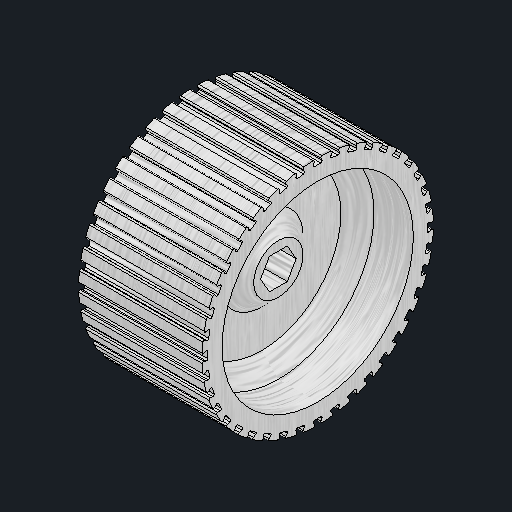
# Autodesk Inventor part: PLATE,FLYWHEEL,HUB
Saved by Autodesk Inventor 2026.1 (Build 301233020, 233B)
## iProperties
Created: 2026-02-01
Part Number: PLATE,FLYWHEEL,HUB
Material: Aluminum 7075
Document SubType Name: Modeling
Designer: Owen L
Mass: 390.303 g
Surface Area: 495.556 cm^2
Volume: 138.898 cm^3
Density: 2.81 g/cm^3
Appearance: Satin - Brushed Heavy
Author: Owen L
Autodesk Inventor part; units mm, degrees
ref_plane "YZ Plane" through (0, 0, 0) normal (1, 0, 0) x (0, 1, 0)
ref_plane "XZ Plane" through (0, 0, 0) normal (0, 1, 0) x (-1, 0, 0)
ref_plane "XY Plane" through (0, 0, 0) normal (0, 0, 1) x (1, 0, 0)
sketch "Sketch1" plane through (0, 0, 0) normal (0, 0, 1) x (1, 0, 0)
  line L0 (0, -9.525) -> (0, 57.15) projected
  line L1 (-35.56, 0) -> (35.56, 0) projected
  line L2 (-9.2075, 0) -> (-9.2075, 10.16)
  line L3 (-9.2075, 10.16) -> (-2.3812, 16.9863)
  line L4 (-2.3812, 16.9863) -> (-2.3813, 32.5438)
  line L5 (-2.3813, 32.5438) -> (-9.2075, 39.37)
  line L6 (-9.2075, 39.37) -> (-25.4, 39.37)
  line L7 (-25.4, 39.37) -> (-25.4, 47.625)
  line L8 (-25.4, 47.625) -> (0, 47.625)
  line L9 (9.2075, 0) -> (9.2075, 10.16)
  line L10 (9.2075, 10.16) -> (2.3812, 16.9863)
  line L11 (2.3812, 16.9863) -> (2.3813, 32.5438)
  line L12 (2.3813, 32.5438) -> (9.2075, 39.37)
  line L13 (9.2075, 39.37) -> (25.4, 39.37)
  line L14 (25.4, 39.37) -> (25.4, 47.625)
  line L15 (25.4, 47.625) -> (0, 47.625)
  point P0 (0, 0)
  dimension "d0" = 10.16
  dimension "d1" = 18.415
  dimension "d3" = 4.7625
  dimension "d4" = 45
  dimension "d5" = 45
  dimension "d6" = 50.8
  dimension "d7" = 8.255
  dimension "d8" = 95.25
  constraints: 28 end point, 7 symmetric about line, 4 perpendicular, 2 point on line, 2 vertical
  measures "d0" distance of L2.start L2.end
  measures "d1" diameter of L2 L0
  measures "d3" diameter of L4 L0
  measures "d4" angle of L1 L3
  measures "d5" angle of L5 L1
  measures "d6" diameter of L7 L0
  measures "d7" distance of L6.end L7.end
  measures "d8" diameter of L8 L1
revolve "Revolution1" add sketch "Sketch1" angle 360 about axis through (-10, 0, 0) along (1, 0, 0)
sketch "Sketch2" plane through (-9.2075, 0, 0) normal (-1, 0, 0) x (0, 0, 1)
  circle A0 centre (0, 0) radius 16.9863 projected
  line L0 (7.3323, 0) -> (3.6662, -6.35)
  line L1 (3.6662, -6.35) -> (-3.6662, -6.35)
  line L2 (-3.6662, -6.35) -> (-7.3323, 0)
  line L3 (-7.3323, 0) -> (-3.6662, 6.35)
  line L4 (-3.6662, 6.35) -> (3.6662, 6.35)
  line L5 (3.6662, 6.35) -> (7.3323, 0)
  dimension "d10" = 12.7
  constraints: 12 end point, 1 coincident, 1 horizontal, 13 other
  measures "d10" distance between parallel lines of L4 L1
extrude "Extrusion1" cut sketch "Sketch2" against normal through all contours L0 L1 L2 L3 L4 L5
sketch "Sketch3" plane through (-25.4, 0, 0) normal (-1, 0, 0) x (0, 0, 1)
  circle A0 centre (0, 0) radius 47.625 projected
  line L0 (-1.016, 47.6142) -> (-2.0955, 45.212)
  line L1 (1.016, 47.6142) -> (2.0955, 45.212)
  line L2 (2.0955, 45.212) -> (-2.0955, 45.212)
  point P0 (0, 45.212)
  dimension "d13" = 4.191
  dimension "d14" = 2.413
  dimension "d15" = 2.032
  constraints: 6 end point, 2 point on circle, 1 equal length, 1 horizontal, 1 midpoint, 1 vertical alignment
  measures "d13" distance of L1.end L0.end
  measures "d14" distance edge to line of A0 L2
  measures "d15" distance of L1.start L0.start
extrude "Extrusion2" cut sketch "Sketch3" against normal through all contours L1 L2 L0 A0 picked at (0.1129, 46.0159)
fillet "Fillet1" radius 0.508 4 edges at (0, 45.212, 2.0955) (0, 45.212, -2.0955) (0, 47.6142, 1.016) (0, 47.6142, -1.016)
pattern_circular "Circular Pattern1" count 40 over 360 about axis through (0, 0, 0) along (1, 0, 0) of "Extrusion2", "Fillet1"
sketch "WaterJet Profile" plane through (0, 0, 0) normal (1, 0, 0) x (0, 1, 0)
  line L0 (55, 55) -> (-55, 55)
  line L1 (-55, 55) -> (-55, -55)
  line L2 (-55, -55) -> (55, -55)
  line L3 (55, -55) -> (55, 55)
  line L4 (55, 55) -> (-55, -55) construction
  line L5 (-55, 55) -> (55, -55) construction
  point P0 (0, 0)
  dimension "d28" = 110
  dimension "d29" = 110
  constraints: 12 end point, 2 midpoint, 2 parallel, 1 horizontal, 1 perpendicular
  measures "d28" distance of L2.end L1.end
  measures "d29" distance of L1.end L0.end
sketch "EDM Profile" plane through (0, 0, 0) normal (1, 0, 0) x (0, 1, 0)
  arc A0 (45.212, -1.3103) -> (45.9282, -1.7736) centre (45.72, -1.3103) ccw projected
  line L0 (45.9282, -1.7736) -> (46.8739, -1.3487) projected
  arc A1 (47.5898, -1.8316) -> (46.8739, -1.3487) centre (47.0821, -1.812) ccw projected
  arc A2 (47.2904, -5.6357) -> (47.5898, -1.8316) centre (0, 0) ccw projected
  arc A3 (46.5078, -6.0006) -> (47.2904, -5.6357) centre (46.7859, -5.5756) ccw projected
  line L1 (46.5078, -6.0006) -> (45.6402, -5.433) projected
  arc A4 (45.6402, -5.433) -> (44.8603, -5.7786) centre (45.3621, -5.858) ccw projected
  line L2 (44.8603, -5.7786) -> (44.4504, -8.3669) projected
  arc A5 (44.4504, -8.3669) -> (45.0853, -8.9366) centre (44.9521, -8.4463) ccw projected
  line L3 (45.0853, -8.9366) -> (46.0858, -8.6647) projected
  arc A6 (46.7173, -9.2537) -> (46.0858, -8.6647) centre (46.219, -9.155) ccw projected
  arc A7 (45.8265, -12.9641) -> (46.7173, -9.2537) centre (0, 0) ccw projected
  arc A8 (44.9965, -13.2022) -> (45.8265, -12.9641) centre (45.3377, -12.8258) ccw projected
  line L4 (44.9965, -13.2022) -> (44.2284, -12.5058) projected
  arc A9 (44.2284, -12.5058) -> (43.4041, -12.7251) centre (43.8872, -12.8821) ccw projected
  line L5 (43.4041, -12.7251) -> (42.5943, -15.2174) projected
  arc A10 (42.5943, -15.2174) -> (43.1323, -15.8794) centre (43.0774, -15.3744) ccw projected
  line L6 (43.1323, -15.8794) -> (44.163, -15.7675) projected
  arc A11 (44.6946, -16.448) -> (44.163, -15.7675) centre (44.2178, -16.2725) ccw projected
  arc A12 (43.2343, -19.9734) -> (44.6946, -16.448) centre (0, 0) ccw projected
  arc A13 (42.3772, -20.0786) -> (43.2343, -19.9734) centre (42.7731, -19.7603) ccw projected
  line L7 (42.3772, -20.0786) -> (41.7276, -19.2707) projected
  arc A14 (41.7276, -19.2707) -> (40.879, -19.3584) centre (41.3317, -19.589) ccw projected
  line L8 (40.879, -19.3584) -> (39.6893, -21.6933) projected
  arc A15 (39.6893, -21.6933) -> (40.1171, -22.4313) centre (40.142, -21.9239) ccw projected
  line L9 (40.1171, -22.4313) -> (41.1527, -22.482) projected
  arc A16 (41.5713, -23.2372) -> (41.1527, -22.482) centre (41.1279, -22.9894) ccw projected
  arc A17 (39.5775, -26.4908) -> (41.5713, -23.2372) centre (0, 0) ccw projected
  arc A18 (38.7145, -26.4607) -> (39.5775, -26.4908) centre (39.1553, -26.2082) ccw projected
  line L10 (38.7145, -26.4607) -> (38.1992, -25.561) projected
  arc A19 (38.1992, -25.561) -> (37.3474, -25.5149) centre (37.7584, -25.8135) ccw projected
  line L11 (37.3474, -25.5149) -> (35.8071, -27.635) projected
  arc A20 (35.8071, -27.635) -> (36.1142, -28.4308) centre (36.2181, -27.9336) ccw projected
  line L12 (36.1142, -28.4308) -> (37.1291, -28.6429) projected
  arc A21 (37.4244, -29.4543) -> (37.1291, -28.6429) centre (37.0252, -29.1401) ccw projected
  arc A22 (34.9462, -32.3559) -> (37.4244, -29.4543) centre (0, 0) ccw projected
  arc A23 (34.0985, -32.1912) -> (34.9462, -32.3559) centre (34.5734, -32.0108) ccw projected
  line L13 (34.0985, -32.1912) -> (33.7303, -31.222) projected
  arc A24 (33.7303, -31.222) -> (32.8962, -31.0432) centre (33.2554, -31.4024) ccw projected
  line L14 (32.8962, -31.0432) -> (31.0432, -32.8962) projected
  arc A25 (31.0432, -32.8962) -> (31.222, -33.7303) centre (31.4024, -33.2554) ccw projected
  line L15 (31.222, -33.7303) -> (32.1912, -34.0985) projected
  arc A26 (32.3559, -34.9462) -> (32.1912, -34.0985) centre (32.0108, -34.5734) ccw projected
  arc A27 (29.4543, -37.4244) -> (32.3559, -34.9462) centre (0, 0) ccw projected
  arc A28 (28.6429, -37.1291) -> (29.4543, -37.4244) centre (29.1401, -37.0252) ccw projected
  line L16 (28.6429, -37.1291) -> (28.4308, -36.1142) projected
  arc A29 (28.4308, -36.1142) -> (27.635, -35.8071) centre (27.9336, -36.2181) ccw projected
  line L17 (27.635, -35.8071) -> (25.5149, -37.3474) projected
  arc A30 (25.5149, -37.3474) -> (25.561, -38.1992) centre (25.8135, -37.7584) ccw projected
  line L18 (25.561, -38.1992) -> (26.4607, -38.7145) projected
  arc A31 (26.4908, -39.5775) -> (26.4607, -38.7145) centre (26.2082, -39.1553) ccw projected
  arc A32 (23.2372, -41.5713) -> (26.4908, -39.5775) centre (0, 0) ccw projected
  arc A33 (22.482, -41.1527) -> (23.2372, -41.5713) centre (22.9894, -41.1279) ccw projected
  line L19 (22.482, -41.1527) -> (22.4313, -40.1171) projected
  arc A34 (22.4313, -40.1171) -> (21.6933, -39.6893) centre (21.9239, -40.142) ccw projected
  line L20 (21.6933, -39.6893) -> (19.3584, -40.879) projected
  arc A35 (19.3584, -40.879) -> (19.2707, -41.7276) centre (19.589, -41.3317) ccw projected
  line L21 (19.2707, -41.7276) -> (20.0786, -42.3772) projected
  arc A36 (19.9734, -43.2343) -> (20.0786, -42.3772) centre (19.7603, -42.7731) ccw projected
  arc A37 (16.448, -44.6946) -> (19.9734, -43.2343) centre (0, 0) ccw projected
  arc A38 (15.7675, -44.163) -> (16.448, -44.6946) centre (16.2725, -44.2178) ccw projected
  line L22 (15.7675, -44.163) -> (15.8794, -43.1323) projected
  arc A39 (15.8794, -43.1323) -> (15.2174, -42.5943) centre (15.3744, -43.0774) ccw projected
  line L23 (15.2174, -42.5943) -> (12.7251, -43.4041) projected
  arc A40 (12.7251, -43.4041) -> (12.5058, -44.2284) centre (12.8821, -43.8872) ccw projected
  line L24 (12.5058, -44.2284) -> (13.2022, -44.9965) projected
  arc A41 (12.9641, -45.8265) -> (13.2022, -44.9965) centre (12.8258, -45.3377) ccw projected
  arc A42 (9.2537, -46.7173) -> (12.9641, -45.8265) centre (0, 0) ccw projected
  arc A43 (8.6647, -46.0858) -> (9.2537, -46.7173) centre (9.155, -46.219) ccw projected
  line L25 (8.6647, -46.0858) -> (8.9366, -45.0853) projected
  arc A44 (8.9366, -45.0853) -> (8.3669, -44.4504) centre (8.4463, -44.9521) ccw projected
  line L26 (8.3669, -44.4504) -> (5.7786, -44.8603) projected
  arc A45 (5.7786, -44.8603) -> (5.433, -45.6402) centre (5.858, -45.3621) ccw projected
  line L27 (5.433, -45.6402) -> (6.0006, -46.5078) projected
  arc A46 (5.6357, -47.2904) -> (6.0006, -46.5078) centre (5.5756, -46.7859) ccw projected
  arc A47 (1.8316, -47.5898) -> (5.6357, -47.2904) centre (0, 0) ccw projected
  arc A48 (1.3487, -46.8739) -> (1.8316, -47.5898) centre (1.812, -47.0821) ccw projected
  line L28 (1.3487, -46.8739) -> (1.7736, -45.9282) projected
  arc A49 (1.7736, -45.9282) -> (1.3103, -45.212) centre (1.3103, -45.72) ccw projected
  line L29 (1.3103, -45.212) -> (-1.3103, -45.212) projected
  arc A50 (-1.3103, -45.212) -> (-1.7736, -45.9282) centre (-1.3103, -45.72) ccw projected
  line L30 (-1.7736, -45.9282) -> (-1.3487, -46.8739) projected
  arc A51 (-1.8316, -47.5898) -> (-1.3487, -46.8739) centre (-1.812, -47.0821) ccw projected
  arc A52 (-5.6357, -47.2904) -> (-1.8316, -47.5898) centre (0, 0) ccw projected
  arc A53 (-6.0006, -46.5078) -> (-5.6357, -47.2904) centre (-5.5756, -46.7859) ccw projected
  line L31 (-6.0006, -46.5078) -> (-5.433, -45.6402) projected
  arc A54 (-5.433, -45.6402) -> (-5.7786, -44.8603) centre (-5.858, -45.3621) ccw projected
  line L32 (-5.7786, -44.8603) -> (-8.3669, -44.4504) projected
  arc A55 (-8.3669, -44.4504) -> (-8.9366, -45.0853) centre (-8.4463, -44.9521) ccw projected
  line L33 (-8.9366, -45.0853) -> (-8.6647, -46.0858) projected
  arc A56 (-9.2537, -46.7173) -> (-8.6647, -46.0858) centre (-9.155, -46.219) ccw projected
  arc A57 (-12.9641, -45.8265) -> (-9.2537, -46.7173) centre (0, 0) ccw projected
  arc A58 (-13.2022, -44.9965) -> (-12.9641, -45.8265) centre (-12.8258, -45.3377) ccw projected
  line L34 (-13.2022, -44.9965) -> (-12.5058, -44.2284) projected
  arc A59 (-12.5058, -44.2284) -> (-12.7251, -43.4041) centre (-12.8821, -43.8872) ccw projected
  line L35 (-12.7251, -43.4041) -> (-15.2174, -42.5943) projected
  arc A60 (-15.2174, -42.5943) -> (-15.8794, -43.1323) centre (-15.3744, -43.0774) ccw projected
  line L36 (-15.8794, -43.1323) -> (-15.7675, -44.163) projected
  arc A61 (-16.448, -44.6946) -> (-15.7675, -44.163) centre (-16.2725, -44.2178) ccw projected
  arc A62 (-19.9734, -43.2343) -> (-16.448, -44.6946) centre (0, 0) ccw projected
  arc A63 (-20.0786, -42.3772) -> (-19.9734, -43.2343) centre (-19.7603, -42.7731) ccw projected
  line L37 (-20.0786, -42.3772) -> (-19.2707, -41.7276) projected
  arc A64 (-19.2707, -41.7276) -> (-19.3584, -40.879) centre (-19.589, -41.3317) ccw projected
  line L38 (-19.3584, -40.879) -> (-21.6933, -39.6893) projected
  arc A65 (-21.6933, -39.6893) -> (-22.4313, -40.1171) centre (-21.9239, -40.142) ccw projected
  line L39 (-22.4313, -40.1171) -> (-22.482, -41.1527) projected
  arc A66 (-23.2372, -41.5713) -> (-22.482, -41.1527) centre (-22.9894, -41.1279) ccw projected
  arc A67 (-26.4908, -39.5775) -> (-23.2372, -41.5713) centre (0, 0) ccw projected
  arc A68 (-26.4607, -38.7145) -> (-26.4908, -39.5775) centre (-26.2082, -39.1553) ccw projected
  line L40 (-26.4607, -38.7145) -> (-25.561, -38.1992) projected
  arc A69 (-25.561, -38.1992) -> (-25.5149, -37.3474) centre (-25.8135, -37.7584) ccw projected
  line L41 (-25.5149, -37.3474) -> (-27.635, -35.8071) projected
  arc A70 (-27.635, -35.8071) -> (-28.4308, -36.1142) centre (-27.9336, -36.2181) ccw projected
  line L42 (-28.4308, -36.1142) -> (-28.6429, -37.1291) projected
  arc A71 (-29.4543, -37.4244) -> (-28.6429, -37.1291) centre (-29.1401, -37.0252) ccw projected
  arc A72 (-32.3559, -34.9462) -> (-29.4543, -37.4244) centre (0, 0) ccw projected
  arc A73 (-32.1912, -34.0985) -> (-32.3559, -34.9462) centre (-32.0108, -34.5734) ccw projected
  line L43 (-32.1912, -34.0985) -> (-31.222, -33.7303) projected
  arc A74 (-31.222, -33.7303) -> (-31.0432, -32.8962) centre (-31.4024, -33.2554) ccw projected
  line L44 (-31.0432, -32.8962) -> (-32.8962, -31.0432) projected
  arc A75 (-32.8962, -31.0432) -> (-33.7303, -31.222) centre (-33.2554, -31.4024) ccw projected
  line L45 (-33.7303, -31.222) -> (-34.0985, -32.1912) projected
  arc A76 (-34.9462, -32.3559) -> (-34.0985, -32.1912) centre (-34.5734, -32.0108) ccw projected
  arc A77 (-37.4244, -29.4543) -> (-34.9462, -32.3559) centre (0, 0) ccw projected
  arc A78 (-37.1291, -28.6429) -> (-37.4244, -29.4543) centre (-37.0252, -29.1401) ccw projected
  line L46 (-37.1291, -28.6429) -> (-36.1142, -28.4308) projected
  arc A79 (-36.1142, -28.4308) -> (-35.8071, -27.635) centre (-36.2181, -27.9336) ccw projected
  line L47 (-35.8071, -27.635) -> (-37.3474, -25.5149) projected
  arc A80 (-37.3474, -25.5149) -> (-38.1992, -25.561) centre (-37.7584, -25.8135) ccw projected
  line L48 (-38.1992, -25.561) -> (-38.7145, -26.4607) projected
  arc A81 (-39.5775, -26.4908) -> (-38.7145, -26.4607) centre (-39.1553, -26.2082) ccw projected
  arc A82 (-41.5713, -23.2372) -> (-39.5775, -26.4908) centre (0, 0) ccw projected
  arc A83 (-41.1527, -22.482) -> (-41.5713, -23.2372) centre (-41.1279, -22.9894) ccw projected
  line L49 (-41.1527, -22.482) -> (-40.1171, -22.4313) projected
  arc A84 (-40.1171, -22.4313) -> (-39.6893, -21.6933) centre (-40.142, -21.9239) ccw projected
  line L50 (-39.6893, -21.6933) -> (-40.879, -19.3584) projected
  arc A85 (-40.879, -19.3584) -> (-41.7276, -19.2707) centre (-41.3317, -19.589) ccw projected
  line L51 (-41.7276, -19.2707) -> (-42.3772, -20.0786) projected
  arc A86 (-43.2343, -19.9734) -> (-42.3772, -20.0786) centre (-42.7731, -19.7603) ccw projected
  arc A87 (-44.6946, -16.448) -> (-43.2343, -19.9734) centre (0, 0) ccw projected
  arc A88 (-44.163, -15.7675) -> (-44.6946, -16.448) centre (-44.2178, -16.2725) ccw projected
  line L52 (-44.163, -15.7675) -> (-43.1323, -15.8794) projected
  arc A89 (-43.1323, -15.8794) -> (-42.5943, -15.2174) centre (-43.0774, -15.3744) ccw projected
  line L53 (-42.5943, -15.2174) -> (-43.4041, -12.7251) projected
  arc A90 (-43.4041, -12.7251) -> (-44.2284, -12.5058) centre (-43.8872, -12.8821) ccw projected
  line L54 (-44.2284, -12.5058) -> (-44.9965, -13.2022) projected
  arc A91 (-45.8265, -12.9641) -> (-44.9965, -13.2022) centre (-45.3377, -12.8258) ccw projected
  arc A92 (-46.7173, -9.2537) -> (-45.8265, -12.9641) centre (0, 0) ccw projected
  arc A93 (-46.0858, -8.6647) -> (-46.7173, -9.2537) centre (-46.219, -9.155) ccw projected
  line L55 (-46.0858, -8.6647) -> (-45.0853, -8.9366) projected
  arc A94 (-45.0853, -8.9366) -> (-44.4504, -8.3669) centre (-44.9521, -8.4463) ccw projected
  line L56 (-44.4504, -8.3669) -> (-44.8603, -5.7786) projected
  arc A95 (-44.8603, -5.7786) -> (-45.6402, -5.433) centre (-45.3621, -5.858) ccw projected
  line L57 (-45.6402, -5.433) -> (-46.5078, -6.0006) projected
  arc A96 (-47.2904, -5.6357) -> (-46.5078, -6.0006) centre (-46.7859, -5.5756) ccw projected
  arc A97 (-47.5898, -1.8316) -> (-47.2904, -5.6357) centre (0, 0) ccw projected
  arc A98 (-46.8739, -1.3487) -> (-47.5898, -1.8316) centre (-47.0821, -1.812) ccw projected
  line L58 (-46.8739, -1.3487) -> (-45.9282, -1.7736) projected
  arc A99 (-45.9282, -1.7736) -> (-45.212, -1.3103) centre (-45.72, -1.3103) ccw projected
  line L59 (-45.212, -1.3103) -> (-45.212, 1.3103) projected
  arc A100 (-45.212, 1.3103) -> (-45.9282, 1.7736) centre (-45.72, 1.3103) ccw projected
  line L60 (-45.9282, 1.7736) -> (-46.8739, 1.3487) projected
  arc A101 (-47.5898, 1.8316) -> (-46.8739, 1.3487) centre (-47.0821, 1.812) ccw projected
  arc A102 (-47.2904, 5.6357) -> (-47.5898, 1.8316) centre (0, 0) ccw projected
  arc A103 (-46.5078, 6.0006) -> (-47.2904, 5.6357) centre (-46.7859, 5.5756) ccw projected
  line L61 (-46.5078, 6.0006) -> (-45.6402, 5.433) projected
  arc A104 (-45.6402, 5.433) -> (-44.8603, 5.7786) centre (-45.3621, 5.858) ccw projected
  line L62 (-44.8603, 5.7786) -> (-44.4504, 8.3669) projected
  arc A105 (-44.4504, 8.3669) -> (-45.0853, 8.9366) centre (-44.9521, 8.4463) ccw projected
  line L63 (-45.0853, 8.9366) -> (-46.0858, 8.6647) projected
  arc A106 (-46.7173, 9.2537) -> (-46.0858, 8.6647) centre (-46.219, 9.155) ccw projected
  arc A107 (-45.8265, 12.9641) -> (-46.7173, 9.2537) centre (0, 0) ccw projected
  arc A108 (-44.9965, 13.2022) -> (-45.8265, 12.9641) centre (-45.3377, 12.8258) ccw projected
  line L64 (-44.9965, 13.2022) -> (-44.2284, 12.5058) projected
  arc A109 (-44.2284, 12.5058) -> (-43.4041, 12.7251) centre (-43.8872, 12.8821) ccw projected
  line L65 (-43.4041, 12.7251) -> (-42.5943, 15.2174) projected
  arc A110 (-42.5943, 15.2174) -> (-43.1323, 15.8794) centre (-43.0774, 15.3744) ccw projected
  line L66 (-43.1323, 15.8794) -> (-44.163, 15.7675) projected
  arc A111 (-44.6946, 16.448) -> (-44.163, 15.7675) centre (-44.2178, 16.2725) ccw projected
  arc A112 (-43.2343, 19.9734) -> (-44.6946, 16.448) centre (0, 0) ccw projected
  arc A113 (-42.3772, 20.0786) -> (-43.2343, 19.9734) centre (-42.7731, 19.7603) ccw projected
  line L67 (-42.3772, 20.0786) -> (-41.7276, 19.2707) projected
  arc A114 (-41.7276, 19.2707) -> (-40.879, 19.3584) centre (-41.3317, 19.589) ccw projected
  line L68 (-40.879, 19.3584) -> (-39.6893, 21.6933) projected
  arc A115 (-39.6893, 21.6933) -> (-40.1171, 22.4313) centre (-40.142, 21.9239) ccw projected
  line L69 (-40.1171, 22.4313) -> (-41.1527, 22.482) projected
  arc A116 (-41.5713, 23.2372) -> (-41.1527, 22.482) centre (-41.1279, 22.9894) ccw projected
  arc A117 (-39.5775, 26.4908) -> (-41.5713, 23.2372) centre (0, 0) ccw projected
  arc A118 (-38.7145, 26.4607) -> (-39.5775, 26.4908) centre (-39.1553, 26.2082) ccw projected
  line L70 (-38.7145, 26.4607) -> (-38.1992, 25.561) projected
  arc A119 (-38.1992, 25.561) -> (-37.3474, 25.5149) centre (-37.7584, 25.8135) ccw projected
  line L71 (-37.3474, 25.5149) -> (-35.8071, 27.635) projected
  arc A120 (-35.8071, 27.635) -> (-36.1142, 28.4308) centre (-36.2181, 27.9336) ccw projected
  line L72 (-36.1142, 28.4308) -> (-37.1291, 28.6429) projected
  arc A121 (-37.4244, 29.4543) -> (-37.1291, 28.6429) centre (-37.0252, 29.1401) ccw projected
  arc A122 (-34.9462, 32.3559) -> (-37.4244, 29.4543) centre (0, 0) ccw projected
  arc A123 (-34.0985, 32.1912) -> (-34.9462, 32.3559) centre (-34.5734, 32.0108) ccw projected
  line L73 (-34.0985, 32.1912) -> (-33.7303, 31.222) projected
  arc A124 (-33.7303, 31.222) -> (-32.8962, 31.0432) centre (-33.2554, 31.4024) ccw projected
  line L74 (-32.8962, 31.0432) -> (-31.0432, 32.8962) projected
  arc A125 (-31.0432, 32.8962) -> (-31.222, 33.7303) centre (-31.4024, 33.2554) ccw projected
  line L75 (-31.222, 33.7303) -> (-32.1912, 34.0985) projected
  arc A126 (-32.3559, 34.9462) -> (-32.1912, 34.0985) centre (-32.0108, 34.5734) ccw projected
  arc A127 (-29.4543, 37.4244) -> (-32.3559, 34.9462) centre (0, 0) ccw projected
  arc A128 (-28.6429, 37.1291) -> (-29.4543, 37.4244) centre (-29.1401, 37.0252) ccw projected
  line L76 (-28.6429, 37.1291) -> (-28.4308, 36.1142) projected
  arc A129 (-28.4308, 36.1142) -> (-27.635, 35.8071) centre (-27.9336, 36.2181) ccw projected
  line L77 (-27.635, 35.8071) -> (-25.5149, 37.3474) projected
  arc A130 (-25.5149, 37.3474) -> (-25.561, 38.1992) centre (-25.8135, 37.7584) ccw projected
  line L78 (-25.561, 38.1992) -> (-26.4607, 38.7145) projected
  arc A131 (-26.4908, 39.5775) -> (-26.4607, 38.7145) centre (-26.2082, 39.1553) ccw projected
  arc A132 (-23.2372, 41.5713) -> (-26.4908, 39.5775) centre (0, 0) ccw projected
  arc A133 (-22.482, 41.1527) -> (-23.2372, 41.5713) centre (-22.9894, 41.1279) ccw projected
  line L79 (-22.482, 41.1527) -> (-22.4313, 40.1171) projected
  arc A134 (-22.4313, 40.1171) -> (-21.6933, 39.6893) centre (-21.9239, 40.142) ccw projected
  line L80 (-21.6933, 39.6893) -> (-19.3584, 40.879) projected
  arc A135 (-19.3584, 40.879) -> (-19.2707, 41.7276) centre (-19.589, 41.3317) ccw projected
  line L81 (-19.2707, 41.7276) -> (-20.0786, 42.3772) projected
  arc A136 (-19.9734, 43.2343) -> (-20.0786, 42.3772) centre (-19.7603, 42.7731) ccw projected
  arc A137 (-16.448, 44.6946) -> (-19.9734, 43.2343) centre (0, 0) ccw projected
  arc A138 (-15.7675, 44.163) -> (-16.448, 44.6946) centre (-16.2725, 44.2178) ccw projected
  line L82 (-15.7675, 44.163) -> (-15.8794, 43.1323) projected
  arc A139 (-15.8794, 43.1323) -> (-15.2174, 42.5943) centre (-15.3744, 43.0774) ccw projected
  line L83 (-15.2174, 42.5943) -> (-12.7251, 43.4041) projected
  arc A140 (-12.7251, 43.4041) -> (-12.5058, 44.2284) centre (-12.8821, 43.8872) ccw projected
  line L84 (-12.5058, 44.2284) -> (-13.2022, 44.9965) projected
  arc A141 (-12.9641, 45.8265) -> (-13.2022, 44.9965) centre (-12.8258, 45.3377) ccw projected
  arc A142 (-9.2537, 46.7173) -> (-12.9641, 45.8265) centre (0, 0) ccw projected
  arc A143 (-8.6647, 46.0858) -> (-9.2537, 46.7173) centre (-9.155, 46.219) ccw projected
  line L85 (-8.6647, 46.0858) -> (-8.9366, 45.0853) projected
  arc A144 (-8.9366, 45.0853) -> (-8.3669, 44.4504) centre (-8.4463, 44.9521) ccw projected
  line L86 (-8.3669, 44.4504) -> (-5.7786, 44.8603) projected
  arc A145 (-5.7786, 44.8603) -> (-5.433, 45.6402) centre (-5.858, 45.3621) ccw projected
  line L87 (-5.433, 45.6402) -> (-6.0006, 46.5078) projected
  arc A146 (-5.6357, 47.2904) -> (-6.0006, 46.5078) centre (-5.5756, 46.7859) ccw projected
  arc A147 (-1.8316, 47.5898) -> (-5.6357, 47.2904) centre (0, 0) ccw projected
  arc A148 (-1.3487, 46.8739) -> (-1.8316, 47.5898) centre (-1.812, 47.0821) ccw projected
  line L88 (-1.3487, 46.8739) -> (-1.7736, 45.9282) projected
  arc A149 (-1.7736, 45.9282) -> (-1.3103, 45.212) centre (-1.3103, 45.72) ccw projected
  line L89 (-1.3103, 45.212) -> (1.3103, 45.212) projected
  arc A150 (1.3103, 45.212) -> (1.7736, 45.9282) centre (1.3103, 45.72) ccw projected
  line L90 (1.7736, 45.9282) -> (1.3487, 46.8739) projected
  arc A151 (1.8316, 47.5898) -> (1.3487, 46.8739) centre (1.812, 47.0821) ccw projected
  arc A152 (5.6357, 47.2904) -> (1.8316, 47.5898) centre (0, 0) ccw projected
  arc A153 (6.0006, 46.5078) -> (5.6357, 47.2904) centre (5.5756, 46.7859) ccw projected
  line L91 (6.0006, 46.5078) -> (5.433, 45.6402) projected
  arc A154 (5.433, 45.6402) -> (5.7786, 44.8603) centre (5.858, 45.3621) ccw projected
  line L92 (5.7786, 44.8603) -> (8.3669, 44.4504) projected
  arc A155 (8.3669, 44.4504) -> (8.9366, 45.0853) centre (8.4463, 44.9521) ccw projected
  line L93 (8.9366, 45.0853) -> (8.6647, 46.0858) projected
  arc A156 (9.2537, 46.7173) -> (8.6647, 46.0858) centre (9.155, 46.219) ccw projected
  arc A157 (12.9641, 45.8265) -> (9.2537, 46.7173) centre (0, 0) ccw projected
  arc A158 (13.2022, 44.9965) -> (12.9641, 45.8265) centre (12.8258, 45.3377) ccw projected
  line L94 (13.2022, 44.9965) -> (12.5058, 44.2284) projected
  arc A159 (12.5058, 44.2284) -> (12.7251, 43.4041) centre (12.8821, 43.8872) ccw projected
  line L95 (12.7251, 43.4041) -> (15.2174, 42.5943) projected
  arc A160 (15.2174, 42.5943) -> (15.8794, 43.1323) centre (15.3744, 43.0774) ccw projected
  line L96 (15.8794, 43.1323) -> (15.7675, 44.163) projected
  arc A161 (16.448, 44.6946) -> (15.7675, 44.163) centre (16.2725, 44.2178) ccw projected
  arc A162 (19.9734, 43.2343) -> (16.448, 44.6946) centre (0, 0) ccw projected
  arc A163 (20.0786, 42.3772) -> (19.9734, 43.2343) centre (19.7603, 42.7731) ccw projected
  line L97 (20.0786, 42.3772) -> (19.2707, 41.7276) projected
  arc A164 (19.2707, 41.7276) -> (19.3584, 40.879) centre (19.589, 41.3317) ccw projected
  line L98 (19.3584, 40.879) -> (21.6933, 39.6893) projected
  arc A165 (21.6933, 39.6893) -> (22.4313, 40.1171) centre (21.9239, 40.142) ccw projected
  line L99 (22.4313, 40.1171) -> (22.482, 41.1527) projected
  arc A166 (23.2372, 41.5713) -> (22.482, 41.1527) centre (22.9894, 41.1279) ccw projected
  arc A167 (26.4908, 39.5775) -> (23.2372, 41.5713) centre (0, 0) ccw projected
  arc A168 (26.4607, 38.7145) -> (26.4908, 39.5775) centre (26.2082, 39.1553) ccw projected
  line L100 (26.4607, 38.7145) -> (25.561, 38.1992) projected
  arc A169 (25.561, 38.1992) -> (25.5149, 37.3474) centre (25.8135, 37.7584) ccw projected
  line L101 (25.5149, 37.3474) -> (27.635, 35.8071) projected
  arc A170 (27.635, 35.8071) -> (28.4308, 36.1142) centre (27.9336, 36.2181) ccw projected
  line L102 (28.4308, 36.1142) -> (28.6429, 37.1291) projected
  arc A171 (29.4543, 37.4244) -> (28.6429, 37.1291) centre (29.1401, 37.0252) ccw projected
  arc A172 (32.3559, 34.9462) -> (29.4543, 37.4244) centre (0, 0) ccw projected
  arc A173 (32.1912, 34.0985) -> (32.3559, 34.9462) centre (32.0108, 34.5734) ccw projected
  line L103 (32.1912, 34.0985) -> (31.222, 33.7303) projected
  arc A174 (31.222, 33.7303) -> (31.0432, 32.8962) centre (31.4024, 33.2554) ccw projected
  line L104 (31.0432, 32.8962) -> (32.8962, 31.0432) projected
  arc A175 (32.8962, 31.0432) -> (33.7303, 31.222) centre (33.2554, 31.4024) ccw projected
  line L105 (33.7303, 31.222) -> (34.0985, 32.1912) projected
  arc A176 (34.9462, 32.3559) -> (34.0985, 32.1912) centre (34.5734, 32.0108) ccw projected
  arc A177 (37.4244, 29.4543) -> (34.9462, 32.3559) centre (0, 0) ccw projected
  arc A178 (37.1291, 28.6429) -> (37.4244, 29.4543) centre (37.0252, 29.1401) ccw projected
  line L106 (37.1291, 28.6429) -> (36.1142, 28.4308) projected
  arc A179 (36.1142, 28.4308) -> (35.8071, 27.635) centre (36.2181, 27.9336) ccw projected
  line L107 (35.8071, 27.635) -> (37.3474, 25.5149) projected
  arc A180 (37.3474, 25.5149) -> (38.1992, 25.561) centre (37.7584, 25.8135) ccw projected
  line L108 (38.1992, 25.561) -> (38.7145, 26.4607) projected
  arc A181 (39.5775, 26.4908) -> (38.7145, 26.4607) centre (39.1553, 26.2082) ccw projected
  arc A182 (41.5713, 23.2372) -> (39.5775, 26.4908) centre (0, 0) ccw projected
  arc A183 (41.1527, 22.482) -> (41.5713, 23.2372) centre (41.1279, 22.9894) ccw projected
  line L109 (41.1527, 22.482) -> (40.1171, 22.4313) projected
  arc A184 (40.1171, 22.4313) -> (39.6893, 21.6933) centre (40.142, 21.9239) ccw projected
  line L110 (39.6893, 21.6933) -> (40.879, 19.3584) projected
  arc A185 (40.879, 19.3584) -> (41.7276, 19.2707) centre (41.3317, 19.589) ccw projected
  line L111 (41.7276, 19.2707) -> (42.3772, 20.0786) projected
  arc A186 (43.2343, 19.9734) -> (42.3772, 20.0786) centre (42.7731, 19.7603) ccw projected
  arc A187 (44.6946, 16.448) -> (43.2343, 19.9734) centre (0, 0) ccw projected
  arc A188 (44.163, 15.7675) -> (44.6946, 16.448) centre (44.2178, 16.2725) ccw projected
  line L112 (44.163, 15.7675) -> (43.1323, 15.8794) projected
  arc A189 (43.1323, 15.8794) -> (42.5943, 15.2174) centre (43.0774, 15.3744) ccw projected
  line L113 (42.5943, 15.2174) -> (43.4041, 12.7251) projected
  arc A190 (43.4041, 12.7251) -> (44.2284, 12.5058) centre (43.8872, 12.8821) ccw projected
  line L114 (44.2284, 12.5058) -> (44.9965, 13.2022) projected
  arc A191 (45.8265, 12.9641) -> (44.9965, 13.2022) centre (45.3377, 12.8258) ccw projected
  arc A192 (46.7173, 9.2537) -> (45.8265, 12.9641) centre (0, 0) ccw projected
  arc A193 (46.0858, 8.6647) -> (46.7173, 9.2537) centre (46.219, 9.155) ccw projected
  line L115 (46.0858, 8.6647) -> (45.0853, 8.9366) projected
  arc A194 (45.0853, 8.9366) -> (44.4504, 8.3669) centre (44.9521, 8.4463) ccw projected
  line L116 (44.4504, 8.3669) -> (44.8603, 5.7786) projected
  arc A195 (44.8603, 5.7786) -> (45.6402, 5.433) centre (45.3621, 5.858) ccw projected
  line L117 (45.6402, 5.433) -> (46.5078, 6.0006) projected
  arc A196 (47.2904, 5.6357) -> (46.5078, 6.0006) centre (46.7859, 5.5756) ccw projected
  arc A197 (47.5898, 1.8316) -> (47.2904, 5.6357) centre (0, 0) ccw projected
  arc A198 (46.8739, 1.3487) -> (47.5898, 1.8316) centre (47.0821, 1.812) ccw projected
  line L118 (46.8739, 1.3487) -> (45.9282, 1.7736) projected
  arc A199 (45.9282, 1.7736) -> (45.212, 1.3103) centre (45.72, 1.3103) ccw projected
  line L119 (45.212, 1.3103) -> (45.212, -1.3103) projected
  line L120 (0, 7.3323) -> (-6.35, 3.6662) projected
  line L121 (-6.35, 3.6662) -> (-6.35, -3.6662) projected
  line L122 (-6.35, -3.6662) -> (0, -7.3323) projected
  line L123 (0, -7.3323) -> (6.35, -3.6662) projected
  line L124 (6.35, -3.6662) -> (6.35, 3.6662) projected
  line L125 (6.35, 3.6662) -> (0, 7.3323) projected
body "Solid1"
